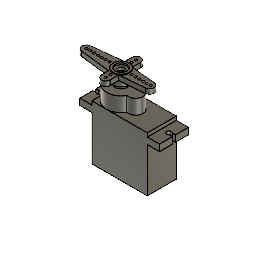
MG90S Micro Servo v2 (Autodesk Fusion 360 design; units mm, degrees)
Autodesk Fusion 360 part; units mm, degrees
sketch "Sketch1" plane through (0, 0, 0) normal (0, 0, 1) x (1, 0, 0)
  line L0 (0, 0) -> (22.8, 0)
  line L1 (22.8, 0) -> (22.8, 12)
  line L2 (22.8, 12) -> (0, 12)
  line L3 (0, 12) -> (0, 0)
  dimension "d1" = 22.8
  dimension "d2" = 12
  constraint coincident L0.start L3.end
  constraint horizontal L0
  constraint perpendicular L0 L1
  constraint perpendicular L1 L2
  constraint perpendicular L0 L3
  measures "d1" distance of L0.start L0.end
  measures "d2" distance of L0.end L1.end
extrude "Extrude1" add sketch "Sketch1" along normal blind 22.5 makes body 1
sketch "Sketch2" plane through (22.8, 0, 0) normal (1, 0, 0) x (0, 1, 0)
  line L0 (0, 0) -> (12, 0)
  line L1 (12, 0) -> (12, 22.5)
  line L2 (12, 22.5) -> (0, 22.5)
  line L3 (0, 22.5) -> (0, 0)
  line L4 (0, 21) -> (12, 21)
  line L5 (12, 21) -> (12, 18.3)
  line L6 (12, 18.3) -> (0, 18.3)
  line L7 (0, 18.3) -> (0, 21)
  dimension "d5" = 1.5
  dimension "d6" = 2.7
  constraint horizontal L4
  constraint vertical L5
  constraint horizontal L6
  constraint vertical L7
  constraint coincident L1 L5.end
  constraint coincident L3 L4.start
  measures "d5" distance of L2.end L4.start
  measures "d6" distance of L4.start L6.end
extrude "Extrude2" add sketch "Sketch2" along normal blind 5 contours L1 L3 L4 L5 L6 L7 bodies 1
sketch "Sketch3" plane through (0, 0, 0) normal (-1, 0, 0) x (0, -1, 0)
  line L0 (-12, 0) -> (0, 0)
  line L1 (0, 0) -> (0, 22.5)
  line L2 (0, 22.5) -> (-12, 22.5)
  line L3 (-12, 22.5) -> (-12, 0)
sketch "Sketch4" plane through (0, 0, 21) normal (0, 0, 1) x (-1, 0, 0)
  line L0 (-22.8, -12) -> (-22.8, 0)
  line L1 (-22.8, 0) -> (-27.8, 0)
  line L2 (-27.8, 0) -> (-27.8, -12)
  line L3 (-27.8, -12) -> (-22.8, -12)
  line L4 (-26.6352, -5.45) -> (-27.8, -5.45)
  line L5 (-26.6352, -6.55) -> (-27.8, -6.55)
  arc A0 (-26.6352, -6.55) -> (-26.6352, -5.45) centre (-25.8, -6) ccw
  line L6 (-27.8, -5.45) -> (-27.8, -6.55)
  dimension "d11" = 2
  dimension "d12" = 2
  constraint horizontal L4
  constraint horizontal L5
  measures "d11" diameter of A0
  measures "d12" horizontal distance of L2.end A0.centre
extrude "Extrude3" cut sketch "Sketch4" against normal blind 2.7 contours L2 L4 L5 A0 L6 bodies 1
ref_plane "WorkPlane1" through (11.4, 6, 9.15) normal (1, 0, 0) x (0, 1, 0)
mirror "Mirror1" about plane through (11.4, 6, 9.15) normal (1, 0, 0) of "Extrude2", "Extrude3"
sketch "Sketch5" plane through (0, 0, 22.5) normal (0, 0, 1) x (-1, 0, 0)
  line L0 (0, -12) -> (0, 0)
  line L1 (0, 0) -> (-22.8, 0)
  line L2 (-22.8, 0) -> (-22.8, -12)
  line L3 (-22.8, -12) -> (0, -12)
  arc A0 (-11.25, -3.0953) -> (-11.25, -8.9047) centre (-12, -6) ccw
  arc A1 (-11.25, -8.9047) -> (-11.25, -3.0953) centre (-6, -6) ccw
  dimension "d18" = 12
  dimension "d19" = 6
  dimension "d20" = 6
  constraint coincident A0.centre A1
  measures "d18" diameter of A1
  measures "d19" horizontal distance of L0.end A1.centre
  measures "d20" diameter of A0
extrude "Extrude4" add sketch "Sketch5" along normal blind 6 contours A0 A1 bodies 1
sketch "Sketch6" plane through (0, 0, 28.5) normal (0, 0, 1) x (-1, 0, 0)
  arc A0 (-11.25, -8.9047) -> (-11.25, -3.0953) centre (-6, -6) ccw
  arc A1 (-11.25, -3.0953) -> (-11.25, -8.9047) centre (-12, -6) ccw
  circle A2 centre (-6, -6) radius 2.45
  dimension "d23" = 4.9
  constraint concentric A0 A2
  measures "d23" diameter of A2
extrude "Extrude5" cut sketch "Sketch6" against normal blind 6 contours A2 bodies 1
copy_body "Body->Comp1" bodies 1 removing the originals makes body 2 in component "MG90S"
sketch "Sketch1 (2)" plane through (0, 0, 22.5) normal (0, 0, 1) x (-1, 0, 0) in component "Servo Spline Axis"
  circle A0 centre (-6, -6) radius 2.45
  circle A1 centre (-6, -6) radius 2.4
  dimension "d26" = 4.8
  constraint concentric A0 A1
  measures "d26" diameter of A1
extrude "Extrude1'" add sketch "Sketch1 (2)" along normal blind 10 separate body contours A1 makes body 3 in component "Servo Spline Axis"
ref_plane "WorkPlane1" through (6, 6, 29.8) normal (0, 0, 1) x (-1, 0, 0) in component "Servo Arm"
sketch "Sketch1 (3)" plane through (6, 6, 29.8) normal (0, 0, 1) x (1, 0, 0) in component "Servo Arm"
  circle A0 centre (0, 0) radius 2.4
  circle A1 centre (0, 0) radius 3.325
  dimension "d43" = 4.8
  dimension "d44" = 6.65
  constraint coincident A0.centre A1.centre
  measures "d43" diameter of A0
  measures "d44" diameter of A1
extrude "Extrude1''" add sketch "Sketch1 (3)" along normal blind 4.5 separate body makes body 4 in component "Servo Arm"
sketch "Sketch2 (2)" plane through (0, 0, 32.5) normal (0, 0, 1) x (-1, 0, 0) in component "Servo Arm"
  circle A0 centre (-6, -6) radius 2.4
  circle A1 centre (-6, -6) radius 2.4
  circle A2 centre (-6, -6) radius 1.25
  dimension "d47" = 4.8
  dimension "d48" = 2.5
  constraint concentric A0 A1
  constraint concentric A1 A2
  measures "d47" diameter of A1
  measures "d48" diameter of A2
extrude "Extrude2'" add sketch "Sketch2 (2)" along normal blind 1.2 bodies 4 in component "Servo Arm"
ref_plane "WorkPlane2" through (6, 6, 34) normal (0, 0, 1) x (1, 0, 0) in component "Servo Arm"
sketch "Sketch3 (2)" plane through (6, 6, 34) normal (0, 0, 1) x (1, 0, 0) in component "Servo Arm"
  line L0 (-1.8, 2.7956) -> (-1.8, 6.3)
  arc A0 (1.8, 6.3) -> (-1.8, 6.3) centre (0, 6.3) ccw
  arc A1 (-1.8, -6.3) -> (1.8, -6.3) centre (0, -6.3) ccw
  line L1 (1.8, -3.35) -> (1.8, -6.3)
  line L2 (-1.8, -2.7956) -> (-1.8, -6.3)
  circle A2 centre (0, 0) radius 3.325
  arc A3 (14.3361, -1.8951) -> (14.3361, 1.8951) centre (14.2, 0) ccw
  line L3 (-1.8, -2.7956) -> (-11.8697, -1.8924)
  line L4 (-1.8, 2.7956) -> (-11.8697, 1.8924)
  arc A4 (-11.8697, 1.8924) -> (-11.8697, -1.8924) centre (-11.7, 0) ccw
  line L5 (1.8, -3.35) -> (14.4188, -1.8874)
  line L6 (1.8, 3.35) -> (14.4188, 1.8874)
  line L7 (1.8, 3.35) -> (1.8, 6.3)
  arc A5 (14.4188, -1.8874) -> (14.4188, 1.8874) centre (14.2, 0) ccw
  circle A6 centre (0, 4.375) radius 0.5
  circle A7 centre (0, 6.175) radius 0.5
  circle A8 centre (0, -4.375) radius 0.5
  circle A9 centre (0, -6.175) radius 0.5
  line L8 (-3.325, 0) -> (-2.4, 0)
  circle A10 centre (-4.4, 0) radius 0.5
  circle A11 centre (-5.96, 0) radius 0.5
  circle A12 centre (-7.52, 0) radius 0.5
  circle A13 centre (-9.08, 0) radius 0.5
  circle A14 centre (-10.64, 0) radius 0.5
  circle A15 centre (-12.2, 0) radius 0.5
  circle A16 centre (4.74, 0) radius 0.5
  circle A17 centre (6.3233, 0) radius 0.5
  circle A18 centre (7.9067, 0) radius 0.5
  circle A19 centre (9.49, 0) radius 0.5
  circle A20 centre (11.0733, 0) radius 0.5
  circle A21 centre (12.6567, 0) radius 0.5
  circle A22 centre (14.24, 0) radius 0.5
  dimension "d52" = 14.2
  dimension "d53" = 6.3
  dimension "d55" = 11.7
  dimension "d58" = 3.8
  dimension "d59" = 6.65
  dimension "d60" = 3.8
  dimension "d62" = 2.95
  dimension "d63" = 2.95
  dimension "d65" = 1
  dimension "d66" = 4.375
  dimension "d68" = 1
  dimension "d69" = 1.8
  dimension "d70" = 1
  dimension "d71" = 2
  dimension "d74" = -7.8
  dimension "d75" = 0
  dimension "d76" = 1
  dimension "d77" = 9.14
  dimension "d80" = 9.5
  dimension "d81" = 0
  constraint coincident A2 L2.start
  constraint tangent L3 A4
  constraint coincident A2 L0.start
  constraint tangent L4 A4
  constraint coincident A3 L5.end
  constraint tangent A3 L5
  constraint concentric A3 A5
  constraint coincident A2 L8.start
  constraint horizontal L8
  measures "d52" distance of A2.centre A3.centre
  measures "d53" distance of A2.centre A0.centre
  measures "d55" distance of A2.centre A4.centre
  measures "d58" diameter of A3
  measures "d59" diameter of A2
  measures "d60" diameter of A4
  measures "d62" vertical distance of A0.centre L6.start
  measures "d63" vertical distance of A1.centre L1.start
  measures "d65" diameter of A6
  measures "d66" distance of A2.centre A6.centre
  measures "d68" diameter of A7
  measures "d69" distance of A6.centre A7.centre
  measures "d70" diameter of A10
  measures "d71" distance of L8.end A10.centre
  measures "d76" diameter of A16
  measures "d77" distance of A10.centre A16.centre
extrude "Extrude3'" add sketch "Sketch3 (2)" against normal blind 2 contours L0 A0 A1 L1 L2 A2 A3 L5 L6 L7 A5 | A2 L3 L4 A4 bodies 4 in component "Servo Arm"
component "MG90S" placed x (1, 0, 0) y (0, 1, 0) z (0, 0, 1) at (0, 0, 0)
component "Servo Spline Axis" placed x (1, 0, 0) y (0, 1, 0) z (0, 0, 1) at (0, 0, 0) in component "MG90S"
component "Servo Arm" placed x (1, 0, 0) y (0, 1, 0) z (0, 0, 1) at (0, 0, 0) in component "MG90S"
equation "d52 = 18 mm - 3.8 mm"
equation "d53 = 8.1 mm - 1.8 mm"
equation "d55 = 15.5 mm - 3.8 mm"
named bodies: "Servo_Case"
